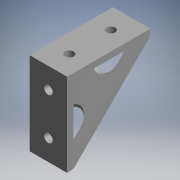
# Autodesk Inventor part: 40-4336 Aluminum
Saved by Autodesk Inventor 2017.3 (Build 213256000, 256)
## iProperties
Part Number: 40-4336 Aluminum
Material: Generic
Catalog Web Link: www.cadenas.de
Description: 25-4136, 40-4336, 30-4366, 45-4366, 25-4136-Black, 40-4336-Black, 30-4366-Black, 45-4366-Black-4 Hole Inside Gusset Corner Bracket
Vendor: 8020
Document SubType Name: Modeling
Designer: partserver
Manufacturer: 8020
Mass: 47.0397 g
Surface Area: 201.138 cm^2
Volume: 47.0397 cm^3
Density: 1 g/cm^3
Appearance: PSOLRGB-191-191-191
Category: PARTsolutions
Company: 8020
Title: 40-4336
Author: Cadenas PARTsolutions
Comments: 4 Hole Inside Gusset Corner Bracket
PSOL_IDENT_0: {$CADENAS_DATA\23d-libs\8020\metric\joining_plates\25_4136.prj},242 {VTYP=3D},{NB=40-4336},{LINA=40-
PSOL_IDENT_1: 4336},{NN=25-4136, 40-4336, 30-4366, 45-4366, 25-4136-Black, 40-4336-Black, 30-4366-Black, 45-4366-B
PSOL_IDENT_2: lack},{DATE=31.07.2020 09:21:28},{GEOMDATE=11.01.2019 21:53:00},{VERSION=},{LINEID=20},{WBVAR=},{WBN
PSOL_IDENT_3: UMERIC=}  {NB=40-4336},{LINA=40-4336},{KT=DUMMY},{PN=40-4336},{SERIES=40},{MATERIAL=Aluminum},{GRADE=
PSOL_IDENT_4: 6105-T5},{FINISH=Clear Anodize},{A=36.00},{B=80.00},{C=80.00},{D=20.00},{E=20.00},{F=8.33},{G=40.00}
PSOL_IDENT_5: ,{T=6.00},{W=.125},{C1=60.000},{C2=20.000},{C3=20.000},{D1=6.000},{COLOR=.75,.75,.75}
NB: 40-4336
NN: 25-4136, 40-4336, 30-4366, 45-4366, 25-4136-Black, 40-4336-Black, 30-4366-Black, 45-4366-Black
NT: 4 Hole Inside Gusset Corner Bracket
NBSYN: $PN.
LINA: 40-4336
CATALOG: 80/20
PN: 40-4336
SERIES: 40
MATERIAL: Aluminum
GRADE: 6105-T5
FINISH: Clear Anodize
A: 36
B: 80
C: 80
D: 20
E: 20
F: 8.33
G: 40
T: 6
W: .125
SUPPLIER: 8020
ARTICLENO: 40-4336
BOMINFO: 40-4336
CREATOR: CADENAS GmbH
Autodesk Inventor part; units mm, degrees
ref_plane "YZ Plane" through (0, 0, 0) normal (1, 0, 0) x (0, 1, 0)
ref_plane "XZ Plane" through (0, 0, 0) normal (0, 1, 0) x (-1, 0, 0)
ref_plane "XY Plane" through (0, 0, 0) normal (0, 0, 1) x (1, 0, 0)
sketch "Sketch_1" plane through (0, 0, 0) normal (1, 0, 0) x (0, 1, 0)
  line L0 (3.5147, 80) -> (0, 80)
  line L1 (0, 80) -> (0, 0)
  line L2 (0, 0) -> (80, 0)
  line L3 (80, 0) -> (80, 3.5147)
  arc A0 (80, 3.5147) -> (78.2426, 7.7574) centre (74, 3.5147) ccw
  line L4 (78.2426, 7.7574) -> (7.7574, 78.2426)
  arc A1 (7.7574, 78.2426) -> (3.5147, 80) centre (3.5147, 74) ccw
  line L5 (6, 71.5147) -> (6, 6)
  line L6 (6, 6) -> (71.5147, 6)
  line L7 (71.5147, 6) -> (6, 71.5147)
  constraints: 16 end point, 4 point on circle, 2 centre point
extrude "Extrusion1" add sketch "Sketch_1" along normal mid plane 36
sketch "Sketch2" plane through (-18, 0, 0) normal (0, -1, 0) x (1, 0, 0)
  point P0 (18, 20)
hole "Hole1" at (0, 0, 20) direction (0, 1, 0) diameter 8.33 depth 6
sketch "Sketch3" plane through (18, 80, 0) normal (0, 0, -1) x (-1, 0, 0)
  point P0 (18, -60)
hole "Hole2" at (0, 20, 0) direction (0, 0, 1) diameter 8.33 depth 6
sketch "Sketch_4" plane through (0, 0, 80) normal (0, 0, 1) x (1, 0, 0)
  circle A0 centre (0, 20) radius 10
  constraints: 1 centre point
extrude "Extrusion2" cut sketch "Sketch_4" against normal blind 74
sketch "Sketch_5" plane through (0, 80, 0) normal (0, 1, 0) x (1, 0, 0)
  circle A0 centre (0, -20) radius 10
  constraints: 1 centre point
extrude "Extrusion3" cut sketch "Sketch_5" against normal blind 74
sketch "Sketch6" plane through (18, 80, 0) normal (0, 0, -1) x (-1, 0, 0)
  point P0 (18, -20)
hole "Hole3" at (0, 60, 0) direction (0, 0, 1) diameter 8.33 depth 6
sketch "Sketch7" plane through (-18, 0, 0) normal (0, -1, 0) x (1, 0, 0)
  point P0 (18, 60)
hole "Hole4" at (0, 0, 60) direction (0, 1, 0) diameter 8.33 depth 6
sketch "Sketch_8" plane through (0, 0, 80) normal (0, 0, 1) x (1, 0, 0)
  circle A0 centre (0, 60) radius 10
  constraints: 1 centre point
extrude "Extrusion4" cut sketch "Sketch_8" against normal blind 74
sketch "Sketch_9" plane through (0, 80, 0) normal (0, 1, 0) x (1, 0, 0)
  circle A0 centre (0, -60) radius 10
  constraints: 1 centre point
extrude "Extrusion5" cut sketch "Sketch_9" against normal blind 74
body "Solid1"
